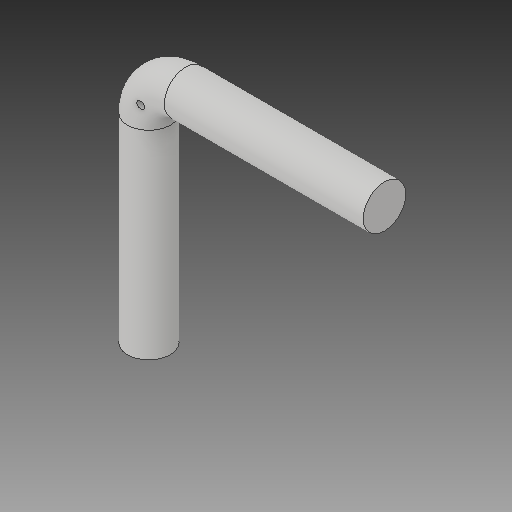
# Autodesk Inventor part: L90roda
Saved by Autodesk Inventor 2018 (Build 220112000, 112)
## iProperties
Created: 2019-12-19
Part Number: L90roda
Material: Generic
Document SubType Name: Modeling
Designer: Ibnu
Density: 1 g/cm^3
Appearance: Default
Author: Ibnu
Autodesk Inventor part; units mm, degrees
ref_plane "XZ Plane" through (0, 0, 0) normal (0, 1, 0) x (-1, 0, 0)
sketch "Sketch1" plane through (0, 0, 0) normal (0, 0, 1) x (1, 0, 0)
  line L0 (25, 0) -> (160, 0)
  line L1 (0, -25) -> (0, -160)
  arc A0 (25, 0) -> (0, -25) centre (25, -25) ccw
  point P0 (0, 0)
  constraints: 4 end point, 2 point on circle, 2 point on line, 2 tangent, 1 centre point, 1 horizontal, 1 vertical
ref_plane "Work Plane1" through (156.75, 0, 0) normal (1, 0, 0) x (0, 1, 0)
sketch "Sketch2" plane through (156.75, 0, 0) normal (1, 0, 0) x (0, 1, 0)
  circle A0 centre (0, 0) radius 14.5
  dimension "d5" = 29
  constraints: 1 centre point, 1 coincident
  measures "d5" diameter of A0
sweep "Sweep1" add profiles "Sketch2" path "Sketch1"
ref_plane "Work Plane2" through (0, 0, 51.25) normal (0, 0, 1) x (1, 0, 0)
sketch "Sketch3" plane through (0, 0, 51.25) normal (0, 0, 1) x (1, 0, 0)
  circle A0 centre (8.7877, -8.7877) radius 2.5
  constraints: 1 centre point
extrude "Extrusion1" cut sketch "Sketch3" against normal through all
body "Solid1"
